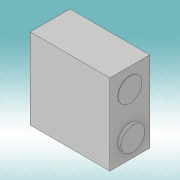
# Autodesk Inventor part: Motor
Saved by Autodesk Inventor 2019 (Build 230136000, 136)
## iProperties
Created: 2019-02-07
Part Number: Motor
Material: Generic
Document SubType Name: Modeling
Designer: USUARIO
Density: 1 g/cm^3
Appearance: Default
Author: USUARIO
Autodesk Inventor part; units mm, degrees
ref_plane "YZ Plane" through (0, 0, 0) normal (1, 0, 0) x (0, 1, 0)
ref_plane "XZ Plane" through (0, 0, 0) normal (0, 1, 0) x (-1, 0, 0)
ref_plane "XY Plane" through (0, 0, 0) normal (0, 0, 1) x (1, 0, 0)
sketch "Sketch1" plane through (0, 0, 0) normal (0, 0, 1) x (1, 0, 0)
  line L0 (0, 0) -> (40, 0)
  line L1 (40, 0) -> (40, -40.5)
  line L2 (40, -40.5) -> (0, -40.5)
  line L3 (0, -40.5) -> (0, 0)
  dimension "d0" = 40
  dimension "d1" = 40.5
  constraints: 8 end point, 2 parallel, 1 horizontal, 1 perpendicular
  measures "d0" distance of L0.start L0.end
  measures "d1" distance of L2.end L0.start
extrude "Extrusion1" add sketch "Sketch1" along normal mid plane 20
sketch "Sketch2" plane through (0, -40.5, 10) normal (-1, 0, 0) x (0, 0, 1)
  line L0 (0, 0) -> (-20, 0) projected
  line L1 (-20, 0) -> (-20, 40.5) projected
  line L2 (0, 40.5) -> (0, 0) projected
  circle A0 centre (-10, 10) radius 6
  line L3 (-20, 20.25) -> (0, 20.25)
  circle A1 centre (-10, 30.5) radius 6
  point P0 (-10, 40.5)
  dimension "d4" = 12
  dimension "d5" = 10
  dimension "d6" = 10
  constraints: 2 centre point, 2 end point, 2 midpoint, 1 horizontal, 1 symmetric about line, 1 other
  measures "d4" diameter of A0
  measures "d5" distance from line of L1 A0.centre
  measures "d6" distance from line of L0 A0.centre
extrude "Extrusion2" add sketch "Sketch2" along normal blind 1.5 contours A0
sketch "Sketch3" plane through (40, -40.5, 10) normal (1, 0, 0) x (0, 0, -1)
  circle A0 centre (10, 10) radius 6 projected
  circle A1 centre (10, 10) radius 6
  line L0 (0, 40.5) -> (0, 0) projected
  line L1 (0, 20.25) -> (20, 20.25)
  line L2 (20, 0) -> (20, 40.5) projected
  circle A2 centre (10, 30.5) radius 6
  point P0 (10, 40.5)
  constraints: 2 centre point, 2 end point, 2 midpoint, 1 coincident, 1 concentric, 1 symmetric about line, 1 other
extrude "Extrusion4" add sketch "Sketch3" along normal blind 1.5 contours A0
extrude "Extrusion5" add sketch "Sketch2" along normal blind 0.1 contours A1
extrude "Extrusion6" add sketch "Sketch3" along normal blind 0.1 contours A2
body "Solid1"
